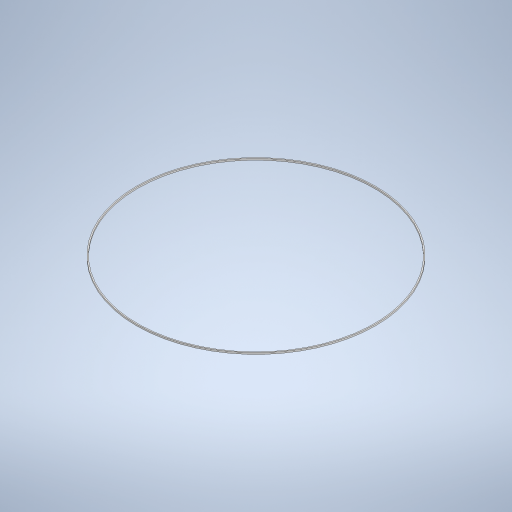
# Autodesk Inventor part: external_diffuser_spacer
Saved by Autodesk Inventor 2024 (Build 280153000, 153)
## iProperties
Created: 2024-01-24
Part Number: external_diffuser_spacer
Material: Generic
Document SubType Name: Modeling
Designer: crow
Density: 1 g/cm^3
Appearance: Default
Author: crow
## iProperties of the stored document external_diffuser_spacer_3DPrint.ipt
Created: 2024-01-24
Part Number: external_diffuser_spacer_3DPrint
Material: Generic
Document SubType Name: Modeling
Designer: crow
Density: 1 g/cm^3
Appearance: Default
Author: crow
Autodesk Inventor part; units mm, degrees
ref_plane "YZ Plane" through (0, 0, 0) normal (1, 0, 0) x (0, 1, 0)
ref_plane "XZ Plane" through (0, 0, 0) normal (0, 1, 0) x (-1, 0, 0)
ref_plane "XY Plane" through (0, 0, 0) normal (0, 0, 1) x (1, 0, 0)
sketch "Sketch1" plane through (0, 0, 0) normal (0, 1, 0) x (-1, 0, 0)
  circle A0 centre (0, 0) radius 90.9
  circle A1 centre (0, 0) radius 90.075
  dimension "d0" = 181.8
  dimension "d1" = 180.15
  constraints: 2 centre point, 2 coincident
  measures "d0" diameter of A0
  measures "d1" diameter of A1
extrude "Extrusion1" add sketch "Sketch1" along normal blind 1.15
body "Solid1"
